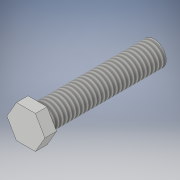
# Autodesk Inventor part: Propeller Bolt
Saved by Autodesk Inventor 2019 (Build 230136000, 136)
## iProperties
Created: 2020-01-19
Part Number: Propeller Bolt
Material: Generic
Document SubType Name: Modeling
Designer: 18186
Density: 1 g/cm^3
Appearance: Default
Author: 18186
Autodesk Inventor part; units mm, degrees
ref_plane "YZ Plane" through (0, 0, 0) normal (1, 0, 0) x (0, 1, 0)
ref_plane "XZ Plane" through (0, 0, 0) normal (0, 1, 0) x (-1, 0, 0)
ref_plane "XY Plane" through (0, 0, 0) normal (0, 0, 1) x (1, 0, 0)
sketch "Sketch1" plane through (0, 0, 0) normal (0, 0, 1) x (1, 0, 0)
  circle A0 centre (0, 0) radius 5.2959
  dimension "d0" = 10.5918
  constraints: 1 centre point, 1 coincident
  measures "d0" diameter of A0
extrude "Extrusion1" add sketch "Sketch1" along normal blind 50.8
sketch "Sketch2" plane through (0, 0, 50.8) normal (0, 0, 1) x (1, 0, 0)
  line L0 (8.2871, 0) -> (4.1435, -7.1768)
  line L1 (4.1435, -7.1768) -> (-4.1435, -7.1768)
  line L2 (-4.1435, -7.1768) -> (-8.2871, 0)
  line L3 (-8.2871, 0) -> (-4.1435, 7.1768)
  line L4 (-4.1435, 7.1768) -> (4.1435, 7.1768)
  line L5 (4.1435, 7.1768) -> (8.2871, 0)
  point P0 (0, 0)
  point P1 (0, 0)
  constraints: 12 end point, 1 coincident, 13 other
extrude "Extrusion2" add sketch "Sketch2" along normal blind 5.08
thread "Thread1" size "7/16-14 UNC" class "2A" standard "ANSI Unified Screw Threads" full length
body "Solid1"
